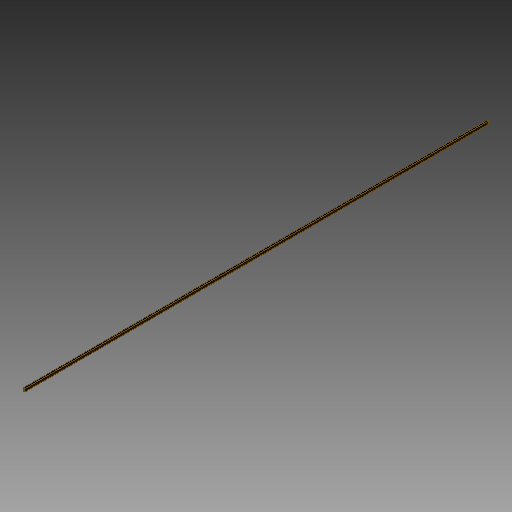
# Autodesk Inventor part: 3216_Rail Brass Track_V1
Saved by Autodesk Inventor 2020 (Build 240168000, 168)
## iProperties
Created: 2019-11-01
Part Number: 3216_Rail Brass Track_V1
Material: Brass, Soft Yellow
Document SubType Name: Modeling
Designer: RFLab
Density: 8.47 g/cm^3
Appearance: Brass - Satin
Mass: 189.816 g
Surface Area: 202.842 cm^2
Volume: 22.4104 cm^3
Author: RFLab
Autodesk Inventor part; units mm, degrees
ref_plane "YZ Plane" through (0, 0, 0) normal (1, 0, 0) x (0, 1, 0)
ref_plane "XZ Plane" through (0, 0, 0) normal (0, 1, 0) x (-1, 0, 0)
ref_plane "XY Plane" through (0, 0, 0) normal (0, 0, 1) x (1, 0, 0)
sketch "Sketch1" plane through (0, 0, 0) normal (0, 0, 1) x (1, 0, 0)
  line L0 (-1.7, -3.175) -> (1.7, -3.175)
  line L1 (1.7, -3.175) -> (1.7, 3.175)
  line L2 (1.7, 3.175) -> (-1.7, 3.175)
  line L3 (-1.7, 3.175) -> (-1.7, -3.175)
  line L4 (-1.7, -3.175) -> (1.7, 3.175) construction
  line L5 (1.7, -3.175) -> (-1.7, 3.175) construction
  point P0 (0, 0)
  dimension "d0" = 3.4
  dimension "d1" = 6.35
  constraints: 12 end point, 2 midpoint, 2 parallel, 1 horizontal, 1 perpendicular
  measures "d0" distance of L2.end L1.end
  measures "d1" distance of L1.end L0.end
extrude "Extrusion1" add sketch "Sketch1" along normal mid plane 1038
body "Solid1"
